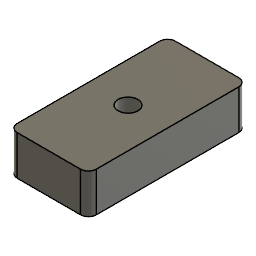
tuturial_block (Autodesk Fusion 360 archive; units mm, degrees)
design "BLOCK"
part number: 2026-07-06-10-52-11-254
Autodesk Fusion 360 part; units mm, degrees
sketch "Sketch1" plane through (0, 0, 0) normal (0, 0, 1) x (1, 0, 0)
  line L0 (0, 0) -> (40, 0)
  line L1 (40, 0) -> (40, -20)
  line L2 (40, -20) -> (0, -20)
  line L3 (0, -20) -> (0, 0)
  constraint horizontal L0
  constraint vertical L1
  constraint horizontal L2
  constraint vertical L3
  constraint coincident L0.start L3.end
sketch "Sketch2" plane through (0, 0, 0) normal (0, 1, 0) x (1, 0, 0)
  line L0 (0, 0) -> (20, 0)
  line L1 (20, 0) -> (20, 40)
  line L2 (20, 40) -> (0, 40)
  line L3 (0, 40) -> (0, 0)
  constraint horizontal L0
  constraint vertical L1
  constraint horizontal L2
  constraint vertical L3
  constraint coincident L0.start L3.end
extrude "Extrude2" add sketch "Sketch2" along normal blind 10
hole "Hole1" at (10, 10, -20) direction (0, -1, 0) diameter 5 depth 10 tip angle 118
fillet "Fillet1" radius 2 1 edges at (20, 5, 0)
fillet "Fillet2" radius 2 1 edges at (0, 5, 0)
fillet "Fillet3" radius 2 1 edges at (0, 5, -40)
fillet "Fillet4" radius 2 1 edges at (20, 5, -40)
